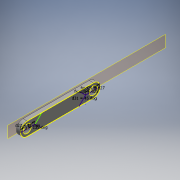
# Autodesk Inventor part: ArmSpan
Saved by Autodesk Inventor 2016 (Build 200138000, 138)
## iProperties
Created: 2016-11-02
Part Number: ArmSpan
Material: Generic
Document SubType Name: Modeling
Designer: mattc
Density: 1 g/cm^3
Appearance: Smooth - Medium Gray
Author: mattc
Autodesk Inventor part; units mm, degrees
ref_plane "YZ Plane" through (0, 0, 0) normal (1, 0, 0) x (0, 1, 0)
ref_plane "XZ Plane" through (0, 0, 0) normal (0, 1, 0) x (-1, 0, 0)
ref_plane "XY Plane" through (0, 0, 0) normal (0, 0, 1) x (1, 0, 0)
sketch "Sketch1" plane through (0, 0, 0) normal (1, 0, 0) x (0, 1, 0)
  circle A0 centre (0, 0) radius 3.1
  arc A1 (0, 5) -> (0, -5) centre (0, 0) ccw
  line L0 (0, 5) -> (50, 5)
  line L1 (50, -5) -> (0, -5)
  arc A2 (50, -5) -> (50, 5) centre (50, 0) ccw
  circle A3 centre (50, 0) radius 3.1
  dimension "d0" = 6.2
  dimension "d1" = 10
  dimension "d3" = 50
  dimension "d5" = 6.2
  dimension "d26" = 5
  constraints: 4 centre point, 4 end point, 4 point on circle, 3 coincident, 3 tangent, 1 horizontal, 1 parallel
  measures "d0" diameter of A0
  measures "d1" diameter of A1
  measures "d3" distance of L0.start L0.end
  measures "d5" diameter of A3
  measures "d26" radius of A2
extrude "Extrusion1" add sketch "Sketch1" along normal blind 3
ref_plane "Work Plane1" through (-2, 0, 0) normal (1, 0, 0) x (0, 0, -1)
sketch "Sketch5" plane through (3, 0, 0) normal (1, 0, 0) x (0, 0, -1)
  line L0 (-5, 50) -> (-5, 0) projected
  arc A0 (-5, 0) -> (5, 0) centre (0, 0) ccw projected
  circle A1 centre (0, 50) radius 3.1 projected
  circle A2 centre (0, 0) radius 3.1 projected
  arc A3 (-5, 0) -> (5, 0) centre (0, 0) ccw projected
  line L1 (5, 0) -> (5, 50) projected
  arc A4 (5, 50) -> (-5, 50) centre (0, 50) ccw projected
  line L2 (-5, 50) -> (-5, 0) projected
  line L3 (0, -5) -> (0, 6)
  line L4 (0, 6) -> (5, 11)
  line L5 (5, 0) -> (5, 50) projected
  line L6 (0, 6) -> (-5, 11)
  line L7 (0, 55) -> (0, 44)
  line L8 (0, 44) -> (-5, 39)
  line L9 (0, 44) -> (5, 39)
  line L10 (0, 44) -> (7.0711, 44) construction
  dimension "d27" = 11
  dimension "d28" = 135
  dimension "d29" = 11
  dimension "d30" = 135
  dimension "d31" = 45
  constraints: 14 end point, 4 point on line, 2 point on circle, 2 vertical, 1 equal length, 1 horizontal
  measures "d27" distance of L3.start L3.end
  measures "d28" angle of L3 L4
  measures "d29" distance of L7.start L7.end
  measures "d30" angle of L7 L8
  measures "d31" angle of L9 L10
equation "\"d5\" = d0"
equation "\"d26\" = 0.5 * d1"
equation "\"d29\" = d27"
equation "\"d30\" = d28"
body "Solid1"
